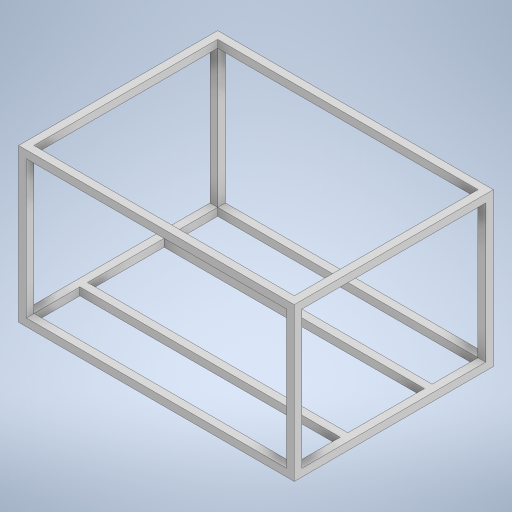
# Autodesk Inventor part: Chassis
Saved by Autodesk Inventor 2023 (Build 270158000, 158)
## iProperties
Created: 2022-08-31
Part Number: Chassis
Material: Generic
Document SubType Name: Modeling
Designer: PC
Density: 1 g/cm^3
Appearance: Default
Author: PC
Autodesk Inventor part; units mm, degrees
ref_plane "YZ Plane" through (0, 0, 0) normal (1, 0, 0) x (0, 1, 0)
ref_plane "XZ Plane" through (0, 0, 0) normal (0, 1, 0) x (-1, 0, 0)
ref_plane "XY Plane" through (0, 0, 0) normal (0, 0, 1) x (1, 0, 0)
sketch "Sketch1" plane through (0, 0, 0) normal (0, 1, 0) x (-1, 0, 0)
  line L0 (457.2, 330.2) -> (-457.2, 330.2)
  line L1 (-457.2, 330.2) -> (-457.2, -330.2)
  line L2 (-457.2, -330.2) -> (457.2, -330.2)
  line L3 (457.2, -330.2) -> (457.2, 330.2)
  line L4 (457.2, 330.2) -> (-457.2, -330.2) construction
  line L5 (-457.2, 330.2) -> (457.2, -330.2) construction
  line L6 (-431.8, -304.8) -> (-431.8, 304.8)
  line L7 (-431.8, 304.8) -> (431.8, 304.8)
  line L8 (431.8, 304.8) -> (431.8, -304.8)
  line L9 (431.8, -304.8) -> (-431.8, -304.8)
  line L10 (-431.8, 152.4) -> (431.8, 152.4)
  line L11 (431.8, 152.4) -> (431.8, 127)
  line L12 (431.8, 127) -> (-431.8, 127)
  line L13 (-431.8, 127) -> (-431.8, 152.4)
  line L14 (431.8, -127) -> (-431.8, -127)
  line L15 (-431.8, -127) -> (-431.8, -152.4)
  line L16 (-431.8, -152.4) -> (431.8, -152.4)
  line L17 (431.8, -152.4) -> (431.8, -127)
  point P0 (0, 0)
  point P1 (0, -152.4)
  dimension "d0" = 914.4
  dimension "d1" = 660.4
  dimension "d2" = 25.4
  dimension "d3" = 25.4
  dimension "d4" = 25.4
  dimension "d5" = 152.4
  dimension "d6" = 152.4
  constraints: 36 end point, 8 parallel, 4 perpendicular, 4 point on line, 3 horizontal, 3 midpoint, 3 other
  measures "d0" distance of L2.end L1.end
  measures "d1" distance of L1.end L0.end
  measures "d2" distance between parallel lines of L1 L6
  measures "d3" distance between parallel lines of L14 L16
  measures "d4" distance between parallel lines of L12 L10
  measures "d5" distance between parallel lines of L7 L10
  measures "d6" distance from line of L9 point (0, -152.4)
extrude "Extrusion1" add sketch "Sketch1" along normal blind 25.4 contours L3 L2 L1 L0 | L6 L14 L8 L16 | L6 L10 L8 L12
sketch "Sketch2" plane through (0, 25.4, 0) normal (0, 1, 0) x (1, 0, 0)
  line L0 (-457.2, 330.2) -> (-457.2, -330.2) projected
  line L1 (431.8, -304.8) -> (-431.8, -304.8) projected
  line L2 (-457.2, -330.2) -> (-431.8, -330.2)
  line L3 (-431.8, -330.2) -> (-431.8, -304.8)
  line L4 (-431.8, -304.8) -> (-457.2, -304.8)
  line L5 (-457.2, -304.8) -> (-457.2, -330.2)
  line L6 (457.2, 330.2) -> (-457.2, 330.2) projected
  line L7 (-431.8, 304.8) -> (431.8, 304.8) projected
  line L8 (-457.2, 330.2) -> (-431.8, 330.2)
  line L9 (-431.8, 330.2) -> (-431.8, 304.8)
  line L10 (-431.8, 304.8) -> (-457.2, 304.8)
  line L11 (-457.2, 304.8) -> (-457.2, 330.2)
  line L12 (457.2, -330.2) -> (457.2, 330.2) projected
  line L13 (457.2, 330.2) -> (431.3742, 330.2)
  line L14 (431.3742, 330.2) -> (431.3742, 304.8)
  line L15 (431.3742, 304.8) -> (457.2, 304.8)
  line L16 (457.2, 304.8) -> (457.2, 330.2)
  line L17 (457.2, -330.2) -> (431.8, -330.2)
  line L18 (431.8, -330.2) -> (431.8, -304.8)
  line L19 (431.8, -304.8) -> (457.2, -304.8)
  line L20 (457.2, -304.8) -> (457.2, -330.2)
  point P0 (0, 0)
  constraints: 32 end point, 8 parallel, 4 horizontal, 4 perpendicular, 3 point on line
extrude "Extrusion2" add sketch "Sketch2" along normal blind 457.2 contours L6 L9 L10 L0 | L4 L3 L2 L0 | L6 L12 L15 L7 L14 | L19 L12 L17 L18
sketch "Sketch3" plane through (0, 482.6, 0) normal (0, 1, 0) x (1, 0, 0)
  line L0 (431.8, -127) -> (-431.8, -127)
  line L1 (-431.8, -127) -> (-431.8, 127)
  line L2 (-431.8, 127) -> (431.8, 127)
  line L3 (431.8, 127) -> (431.8, -127)
  line L4 (457.2, 304.8) -> (431.8, 304.8)
  line L5 (431.8, 304.8) -> (431.8, 152.4)
  line L6 (431.8, 152.4) -> (-431.8, 152.4)
  line L7 (-431.8, 152.4) -> (-431.8, 304.8)
  line L8 (-431.8, 304.8) -> (-457.2, 304.8)
  line L9 (-457.2, 304.8) -> (-457.2, -304.8)
  line L10 (-457.2, -304.8) -> (-431.8, -304.8)
  line L11 (-431.8, -304.8) -> (-431.8, -152.4)
  line L12 (-431.8, -152.4) -> (431.8, -152.4)
  line L13 (431.8, -152.4) -> (431.8, -304.8)
  line L14 (431.8, -304.8) -> (457.2, -304.8)
  line L15 (457.2, -304.8) -> (457.2, 304.8)
  line L16 (431.3742, 304.8) -> (431.3742, 330.2)
  line L17 (431.3742, 330.2) -> (-431.8, 330.2)
  line L18 (-431.8, 330.2) -> (-431.8, 304.8)
  line L19 (-431.8, 304.8) -> (431.3742, 304.8)
  line L20 (431.8, -330.2) -> (431.8, -304.8)
  line L21 (431.8, -304.8) -> (-431.8, -304.8)
  line L22 (-431.8, -304.8) -> (-431.8, -330.2)
  line L23 (-431.8, -330.2) -> (431.8, -330.2)
  line L24 (-431.8, -330.2) -> (-431.8, -304.8)
  line L25 (-431.8, -304.8) -> (-457.2, -304.8)
  line L26 (-457.2, -304.8) -> (-457.2, -330.2)
  line L27 (-457.2, -330.2) -> (-431.8, -330.2)
  line L28 (-431.8, 304.8) -> (-431.8, 330.2)
  line L29 (-431.8, 330.2) -> (-457.2, 330.2)
  line L30 (-457.2, 330.2) -> (-457.2, 304.8)
  line L31 (-457.2, 304.8) -> (-431.8, 304.8)
  line L32 (457.2, 304.8) -> (457.2, 330.2)
  line L33 (457.2, 330.2) -> (431.3742, 330.2)
  line L34 (431.3742, 330.2) -> (431.3742, 304.8)
  line L35 (431.3742, 304.8) -> (457.2, 304.8)
  line L36 (457.2, -304.8) -> (431.8, -304.8)
  line L37 (431.8, -330.2) -> (457.2, -330.2)
  line L38 (457.2, -330.2) -> (457.2, -304.8)
  line L39 (457.2, -304.8) -> (431.8, -304.8)
  line L40 (431.8, -304.8) -> (431.8, -330.2)
  line L41 (431.8, -152.4) -> (431.8, -304.8)
  line L42 (431.8, -152.4) -> (431.8, 152.4)
  line L43 (431.8, 127) -> (431.8, -127)
  line L44 (-431.8, -152.4) -> (-431.8, 152.4)
  point P0 (0, 0)
  point P1 (431.8, 127)
extrude "Extrusion3" add sketch "Sketch3" along normal blind 25.4 contours L3 L42 L5 L4 L15 L14 L13 | L44 L11 L10 L9 L8 L7 L1 | L14 L38 L37 L20 | L20 L23 L22 L21 | L22 L27 L26 L10 | L35 L16 L33 L32 L4 | L8 L30 L29 L18 | L18 L17 L16 L19
equation "\"d6\" = d5"
body "Solid1"
